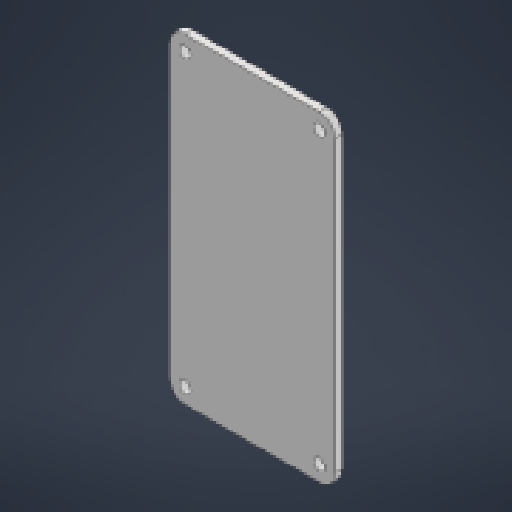
# Autodesk Inventor part: esp_plate
Saved by Autodesk Inventor 2024 (Build 280153000, 153)
## iProperties
Created: 2026-03-25
Part Number: esp_plate
Material: Generic
Document SubType Name: Modeling
Designer: schar
Density: 1 g/cm^3
Appearance: Default
Author: schar
Autodesk Inventor part; units mm, degrees
ref_plane "YZ Plane" through (0, 0, 0) normal (1, 0, 0) x (0, 1, 0)
ref_plane "XZ Plane" through (0, 0, 0) normal (0, 1, 0) x (-1, 0, 0)
ref_plane "XY Plane" through (0, 0, 0) normal (0, 0, 1) x (1, 0, 0)
sketch "Sketch1" plane through (0, 0, 0) normal (0, 0, 1) x (1, 0, 0)
  circle A0 centre (0, 0) radius 4
  circle A1 centre (35, 0) radius 1.5 projected
  circle A2 centre (35, -75.4552) radius 1.5 projected
  circle A3 centre (0, -75.4552) radius 1.5 projected
  circle A4 centre (35, 0) radius 4
  circle A5 centre (0, -75.4552) radius 4
  circle A6 centre (35, -75.4552) radius 4
  circle A7 centre (0, 0) radius 1.5
  line L0 (0, 4) -> (35, 4)
  line L1 (39, 0) -> (39, -75.4552)
  line L2 (35, -79.4552) -> (0, -79.4552)
  line L3 (-4, -75.4552) -> (-4, 0)
  dimension "d0" = 8
  dimension "d1" = 8
  dimension "d2" = 8
  dimension "d3" = 8
  dimension "d4" = 3
  constraints: 8 end point, 8 point on circle, 5 centre point, 5 coincident, 5 tangent, 1 horizontal
  measures "d0" diameter of A0
  measures "d1" diameter of A4
  measures "d2" diameter of A5
  measures "d3" diameter of A6
  measures "d4" diameter of A7
extrude "Extrusion1" add sketch "Sketch1" along normal blind 2
sketch "Sketch2" plane through (0, 0, 0) normal (0, 0, -1) x (-1, 0, 0)
  line L0 (-35, 4) -> (0, 4) projected
  line L1 (4, 0) -> (4, -75.4552) projected
  line L2 (4, -37.7276) -> (-25.3543, -37.7276)
  line L3 (-34.5, -6.7276) -> (-7.5, -6.7276)
  line L4 (-7.5, -6.7276) -> (-7.5, -68.7276)
  line L5 (-7.5, -68.7276) -> (-34.5, -68.7276)
  line L6 (-34.5, -68.7276) -> (-34.5, -6.7276)
  line L7 (-34.5, -6.7276) -> (-7.5, -68.7276) construction
  line L8 (-7.5, -6.7276) -> (-34.5, -68.7276) construction
  line L9 (-39, -75.4552) -> (-39, 0) projected
  point P0 (0, 0)
  point P1 (-21, -37.7276)
  point P2 (-39, -37.7276)
  dimension "d7" = 27
  dimension "d8" = 62
  dimension "d12" = 18
  constraints: 14 end point, 4 midpoint, 2 horizontal, 2 parallel, 1 perpendicular, 1 point on line
  measures "d7" distance of L4.end L5.end
  measures "d8" distance of L3.end L4.end
  measures "d12" distance of point (-39, -37.728) point (-21, -37.728)
extrude "Extrusion2" add sketch "Sketch2" along normal blind 4
body "Solid1"
